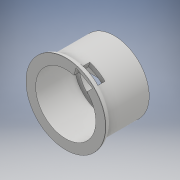
# Autodesk Inventor part: BaseRod_Pepu
Saved by Autodesk Inventor 2018 (Build 220112000, 112)
## iProperties
Created: 2020-11-14
Part Number: BaseRod_Pepu
Material: Genérico
Document SubType Name: Modeling
Designer: orgyn
Density: 1 g/cm^3
Appearance: Valor por defecto
Author: orgyn
Autodesk Inventor part; units mm, degrees
ref_plane "YZ Plane" through (0, 0, 0) normal (1, 0, 0) x (0, 1, 0)
ref_plane "XZ Plane" through (0, 0, 0) normal (0, 1, 0) x (-1, 0, 0)
ref_plane "XY Plane" through (0, 0, 0) normal (0, 0, 1) x (1, 0, 0)
sketch "Boceto1" plane through (0, 0, 0) normal (0, 1, 0) x (-1, 0, 0)
  circle A0 centre (0, 0) radius 62
  circle A1 centre (0, 0) radius 72
  circle A2 centre (0, 0) radius 52
  dimension "d5" = 124
  dimension "d6" = 144
  dimension "d7" = 104
  constraints: 3 centre point, 3 coincident
  measures "d5" diameter of A0
  measures "d6" diameter of A1
  measures "d7" diameter of A2
extrude "Extrusión1" add sketch "Boceto1" along normal blind 100 contours A1
sketch "Boceto5" plane through (0, 0, 0) normal (0, -1, 0) x (1, 0, 0)
  circle A0 centre (0, 0) radius 52
  circle A1 centre (0, 0) radius 62
  dimension "d11" = 104
  dimension "d12" = 124
  constraints: 2 centre point, 2 coincident
  measures "d11" diameter of A0
  measures "d12" diameter of A1
extrude "Extrusión2" add sketch "Boceto5" against normal blind 95
sketch "Boceto6" plane through (0, 0, 0) normal (0, -1, 0) x (1, 0, 0)
  circle A0 centre (0, 0) radius 52
  circle A1 centre (0, 0) radius 62
  dimension "d15" = 104
  dimension "d16" = 124
  constraints: 2 centre point, 2 coincident
  measures "d15" diameter of A0
  measures "d16" diameter of A1
extrude "Extrusión3" cut sketch "Boceto6" against normal blind 80
sketch "Boceto7" plane through (0, 0, 0) normal (0, -1, 0) x (1, 0, 0)
  circle A0 centre (0, 0) radius 82
  circle A1 centre (0, 0) radius 72
  dimension "d19" = 164
  dimension "d20" = 144
  constraints: 2 centre point, 2 coincident
  measures "d19" diameter of A0
  measures "d20" diameter of A1
extrude "Extrusión4" add sketch "Boceto7" against normal blind 15
fillet "Empalme1" radius 15 1 edges at (-82, 15, 0)
sketch "Boceto8" plane through (0, 0, 0) normal (0, -1, 0) x (1, 0, 0)
  arc A0 (43.8491, 43.8321) -> (16.8777, 59.6586) centre (0, 0) ccw
  line L0 (43.8491, 43.8321) -> (50.9216, 50.9018)
  line L1 (16.8777, 59.6586) -> (19.5999, 69.2809)
  line L2 (19.5999, 69.2809) -> (21.3442, 75.4464)
  line L3 (21.3442, 75.4464) -> (55.4532, 55.4317)
  line L4 (55.4532, 55.4317) -> (50.9216, 50.9018)
  dimension "d25" = 124
  constraints: 10 end point, 2 point on circle, 1 centre point
  measures "d25" diameter of A0
extrude "Extrusión5" cut sketch "Boceto8" against normal blind 30
sketch "Boceto9" plane through (0, 95, 0) normal (0, 1, 0) x (1, 0, 0)
  line L0 (51.775, -4.7614) -> (51.775, 6.1116)
  line L1 (5.2843, 55.289) -> (-4.7157, 55.289)
  line L2 (5.2843, 55.289) -> (5.2843, -56.0708)
  line L3 (5.2843, -56.0708) -> (-4.7157, -56.0708)
  line L4 (-4.7157, -56.0708) -> (-4.7157, 55.289)
  line L5 (5.2843, 55.289) -> (-4.7157, 55.289)
  line L6 (5.2843, 55.289) -> (5.2843, -56.0708)
  line L7 (5.2843, -56.0708) -> (-4.7157, -56.0708)
  line L8 (-4.7157, -56.0708) -> (-4.7157, 55.289)
  line L9 (-56.1571, 4.9777) -> (-56.1571, -5.0223)
  line L10 (-56.1571, 4.9777) -> (55.2027, 4.9777)
  line L11 (55.2027, 4.9777) -> (55.2027, -5.0223)
  line L12 (55.2027, -5.0223) -> (-56.1571, -5.0223)
  constraints: 26 end point, 6 perpendicular
extrude "Extrusión6" cut sketch "Boceto9" against normal blind 10
sketch "Boceto10" plane through (0, 85, 0) normal (0, 1, 0) x (1, 0, 0)
  line L0 (-51.7569, -5.0223) -> (-56.1571, -5.0223) projected
  line L1 (55.2027, -5.0223) -> (51.7569, -5.0223) projected
  line L2 (-56.1571, -5.0223) -> (55.2027, -5.0223)
  line L3 (55.2027, -5.0223) -> (55.2027, 4.9777)
  line L4 (-56.1571, 4.9777) -> (-51.7612, 4.9777) projected
  line L5 (55.2027, 4.9777) -> (-56.1571, 4.9777)
  line L6 (-56.1571, -5.0223) -> (-56.1571, 4.9777) projected
  line L7 (-56.1571, 4.9777) -> (-56.1571, -5.0223)
  line L8 (-4.7157, -56.0708) -> (-4.7157, -51.7857) projected
  line L9 (5.2843, -56.0708) -> (-4.7157, -56.0708) projected
  line L10 (-4.7157, -56.0708) -> (5.2843, -56.0708)
  line L11 (5.2843, 55.289) -> (5.2843, 51.7308) projected
  line L12 (5.2843, -56.0708) -> (5.2843, 55.289)
  line L13 (-4.7157, 55.289) -> (5.2843, 55.289) projected
  line L14 (5.2843, 55.289) -> (-4.7157, 55.289)
  line L15 (-4.7157, 55.289) -> (-4.7157, -56.0708)
  point P0 (0, 0)
  constraints: 16 end point, 5 perpendicular, 2 horizontal, 1 collinear
extrude "Extrusión7" add sketch "Boceto10" along normal blind 8
sketch "Boceto11" plane through (0, 85, 0) normal (0, -1, 0) x (1, 0, 0)
  line L0 (0, 0) -> (0, -9.6645)
  constraints: 2 end point, 1 vertical
